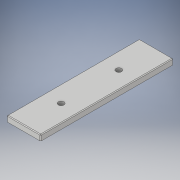
# Autodesk Inventor part: Carrier
Saved by Autodesk Inventor 2019.4 (Build 234330000, 330)
## iProperties
Created: 2021-04-21
Part Number: Carrier
Material: Generic
Document SubType Name: Modeling
Designer: caleb
Density: 1 g/cm^3
Appearance: Default
Author: caleb
Autodesk Inventor part; units mm, degrees
ref_plane "YZ Plane" through (0, 0, 0) normal (1, 0, 0) x (0, 1, 0)
ref_plane "XZ Plane" through (0, 0, 0) normal (0, 1, 0) x (-1, 0, 0)
ref_plane "XY Plane" through (0, 0, 0) normal (0, 0, 1) x (1, 0, 0)
sketch "Sketch1" plane through (0, 0, 0) normal (0, 1, 0) x (-1, 0, 0)
  line L0 (-19.05, 74.6125) -> (19.05, 74.6125)
  line L1 (19.05, 74.6125) -> (19.05, -74.6125)
  line L2 (19.05, -74.6125) -> (-19.05, -74.6125)
  line L3 (-19.05, -74.6125) -> (-19.05, 74.6125)
  line L4 (-19.05, 74.6125) -> (19.05, -74.6125) construction
  line L5 (19.05, 74.6125) -> (-19.05, -74.6125) construction
  point P0 (0, 0)
  dimension "d0" = 149.225
  dimension "d1" = 38.1
  constraints: 12 end point, 2 midpoint, 2 parallel, 1 horizontal, 1 perpendicular
  measures "d0" distance of L0.end L1.end
  measures "d1" distance of L1.end L2.end
extrude "Extrusion1" add sketch "Sketch1" along normal blind 6.35
sketch "Sketch2" plane through (0, 6.35, 0) normal (0, 1, 0) x (1, 0, 0)
  point P0 (0, 0)
  point P1 (0, -32.5)
  point P2 (0, 32.5)
  dimension "d4" = 32.5
  dimension "d5" = 32.5
  measures "d4" distance of point (0, 0) point (0, -32.5)
  measures "d5" distance of point (0, 0) point (0, 32.5)
hole "Hole1" at (0, 6.35, 32.5) at (0, 6.35, -32.5) direction (0, -1, 0) diameter 6.35 end through all
chamfer "Chamfer1" distance 0.7937 angle 45 8 edges at (19.05, 6.35, 0) (0, 6.35, 74.6125) (0, 6.35, -74.6125) (-19.05, 6.35, 0) (-19.05, 3.175, -74.6125) (19.05, 3.175, -74.6125) (-19.05, 3.175, 74.6125) (19.05, 3.175, 74.6125)
body "Solid1"
